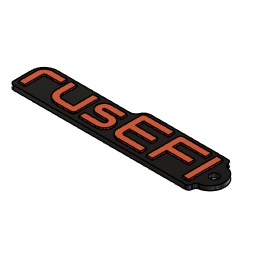
rusEFI Key chain v7 (Autodesk Fusion 360 design; units mm, degrees)
Autodesk Fusion 360 part; units mm, degrees
note: some values were not read from the file. Chosen so that the rebuilt part matches the saved one: which bodies a step acts on.
sketch "Sketch1" plane through (0, 0, 0) normal (0, 0, 1) x (1, 0, 0)
  line L0 (13.2775, 11.4505) -> (5.1185, 11.4505)
  spline S0 degree 2 poles (5.1185, 11.4505) (4.3794, 11.4505) (4.0028, 11.0809) knots 0 0 0 1 1 1
  spline S1 degree 2 poles (4.0028, 11.0809) (3.6262, 10.7113) (3.6262, 10) knots 0 0 0 1 1 1
  line L1 (3.6262, 10) -> (3.6262, 0)
  line L2 (3.6262, 0) -> (0, 0)
  line L3 (0, 0) -> (0, 10)
  spline S2 degree 2 poles (0, 10) (0, 10.9344) (0.2371, 11.6736) knots 0 0 0 1 1 1
  spline S3 degree 2 poles (0.2371, 11.6736) (0.4742, 12.4128) (0.8717, 12.9777) knots 0 0 0 1 1 1
  spline S4 degree 2 poles (0.8717, 12.9777) (1.2692, 13.5425) (1.7852, 13.94) knots 0 0 0 1 1 1
  spline S5 degree 2 poles (1.7852, 13.94) (2.3013, 14.3375) (2.8661, 14.5886) knots 0 0 0 1 1 1
  spline S6 degree 2 poles (2.8661, 14.5886) (3.431, 14.8396) (4.0098, 14.9582) knots 0 0 0 1 1 1
  spline S7 degree 2 poles (4.0098, 14.9582) (4.5886, 15.0767) (5.0907, 15.0767) knots 0 0 0 1 1 1
  line L4 (5.0907, 15.0767) -> (13.2775, 15.0767)
  line L5 (13.2775, 15.0767) -> (13.2775, 11.4505)
  spline S8 degree 2 poles (32.1478, 1.8271) (32.1478, 1.4365) (32.0084, 1.1018) knots 0 0 0 1 1 1
  spline S9 degree 2 poles (32.0084, 1.1018) (31.8689, 0.7671) (31.6248, 0.523) knots 0 0 0 1 1 1
  spline S10 degree 2 poles (31.6248, 0.523) (31.3808, 0.2789) (31.053, 0.1395) knots 0 0 0 1 1 1
  spline S11 degree 2 poles (31.053, 0.1395) (30.7252, 0) (30.3487, 0) knots 0 0 0 1 1 1
  line L6 (30.3487, 0) -> (22.1478, 0)
  spline S12 degree 2 poles (22.1478, 0) (21.4784, 0) (20.7183, 0.1534) knots 0 0 0 1 1 1
  spline S13 degree 2 poles (20.7183, 0.1534) (19.9582, 0.3068) (19.219, 0.6485) knots 0 0 0 1 1 1
  spline S14 degree 2 poles (19.219, 0.6485) (18.4798, 0.9902) (17.7894, 1.5132) knots 0 0 0 1 1 1
  spline S15 degree 2 poles (17.7894, 1.5132) (17.099, 2.0363) (16.583, 2.7824) knots 0 0 0 1 1 1
  spline S16 degree 2 poles (16.583, 2.7824) (16.0669, 3.5286) (15.7531, 4.5049) knots 0 0 0 1 1 1
  spline S17 degree 2 poles (15.7531, 4.5049) (15.4393, 5.4812) (15.4393, 6.7085) knots 0 0 0 1 1 1
  line L7 (15.4393, 6.7085) -> (15.4393, 15.0767)
  line L8 (15.4393, 15.0767) -> (19.0656, 15.0767)
  line L9 (19.0656, 15.0767) -> (19.0656, 6.7085)
  spline S18 degree 2 poles (19.0656, 6.7085) (19.0656, 5.9972) (19.3096, 5.4324) knots 0 0 0 1 1 1
  spline S19 degree 2 poles (19.3096, 5.4324) (19.5537, 4.8675) (19.9721, 4.463) knots 0 0 0 1 1 1
  spline S20 degree 2 poles (19.9721, 4.463) (20.3905, 4.0586) (20.9554, 3.8424) knots 0 0 0 1 1 1
  spline S21 degree 2 poles (20.9554, 3.8424) (21.5202, 3.6262) (22.1757, 3.6262) knots 0 0 0 1 1 1
  line L10 (22.1757, 3.6262) -> (28.5216, 3.6262)
  line L11 (28.5216, 3.6262) -> (28.5216, 15.0767)
  line L12 (28.5216, 15.0767) -> (32.1478, 15.0767)
  line L13 (32.1478, 15.0767) -> (32.1478, 1.8271)
  spline S22 degree 2 poles (50.1255, 5.0907) (50.1255, 4.1562) (49.8884, 3.41) knots 0 0 0 1 1 1
  spline S23 degree 2 poles (49.8884, 3.41) (49.6513, 2.6639) (49.2608, 2.099) knots 0 0 0 1 1 1
  spline S24 degree 2 poles (49.2608, 2.099) (48.8703, 1.5342) (48.3543, 1.1367) knots 0 0 0 1 1 1
  spline S25 degree 2 poles (48.3543, 1.1367) (47.8382, 0.7392) (47.2734, 0.4881) knots 0 0 0 1 1 1
  spline S26 degree 2 poles (47.2734, 0.4881) (46.7085, 0.2371) (46.1297, 0.1186) knots 0 0 0 1 1 1
  spline S27 degree 2 poles (46.1297, 0.1186) (45.5509, 0) (45.0349, 0) knots 0 0 0 1 1 1
  line L14 (45.0349, 0) -> (35.2162, 0)
  line L15 (35.2162, 0) -> (35.2162, 3.6262)
  line L16 (35.2162, 3.6262) -> (45.007, 3.6262)
  spline S28 degree 2 poles (45.007, 3.6262) (45.7462, 3.6262) (46.1227, 4.0028) knots 0 0 0 1 1 1
  spline S29 degree 2 poles (46.1227, 4.0028) (46.4993, 4.3794) (46.4993, 5.0907) knots 0 0 0 1 1 1
  spline S30 degree 2 poles (46.4993, 5.0907) (46.4296, 6.5411) (45.0349, 6.5411) knots 0 0 0 1 1 1
  line L17 (45.0349, 6.5411) -> (39.4142, 6.5411)
  spline S31 degree 2 poles (39.4142, 6.5411) (38.2148, 6.5411) (37.378, 6.9596) knots 0 0 0 1 1 1
  spline S32 degree 2 poles (37.378, 6.9596) (36.5411, 7.378) (36.0181, 8.0056) knots 0 0 0 1 1 1
  spline S33 degree 2 poles (36.0181, 8.0056) (35.4951, 8.6332) (35.265, 9.3584) knots 0 0 0 1 1 1
  spline S34 degree 2 poles (35.265, 9.3584) (35.0349, 10.0837) (35.0349, 10.7113) knots 0 0 0 1 1 1
  spline S35 degree 2 poles (35.0349, 10.7113) (35.0349, 11.9247) (35.4672, 12.7545) knots 0 0 0 1 1 1
  spline S36 degree 2 poles (35.4672, 12.7545) (35.8996, 13.5844) (36.5551, 14.1004) knots 0 0 0 1 1 1
  spline S37 degree 2 poles (36.5551, 14.1004) (37.2106, 14.6165) (37.9777, 14.8466) knots 0 0 0 1 1 1
  spline S38 degree 2 poles (37.9777, 14.8466) (38.7448, 15.0767) (39.4142, 15.0767) knots 0 0 0 1 1 1
  line L18 (39.4142, 15.0767) -> (48.3264, 15.0767)
  line L19 (48.3264, 15.0767) -> (48.3264, 11.4505)
  line L20 (48.3264, 11.4505) -> (39.4421, 11.4505)
  spline S39 degree 2 poles (39.4421, 11.4505) (39.1632, 11.4505) (39.0028, 11.3877) knots 0 0 0 1 1 1
  spline S40 degree 2 poles (39.0028, 11.3877) (38.8424, 11.325) (38.7657, 11.2204) knots 0 0 0 1 1 1
  spline S41 degree 2 poles (38.7657, 11.2204) (38.689, 11.1158) (38.675, 10.9972) knots 0 0 0 1 1 1
  spline S42 degree 2 poles (38.675, 10.9972) (38.6611, 10.8787) (38.6611, 10.7671) knots 0 0 0 1 1 1
  spline S43 degree 2 poles (38.6611, 10.7671) (38.675, 10.5439) (38.7448, 10.4184) knots 0 0 0 1 1 1
  spline S44 degree 2 poles (38.7448, 10.4184) (38.8145, 10.2929) (38.9191, 10.2371) knots 0 0 0 1 1 1
  spline S45 degree 2 poles (38.9191, 10.2371) (39.0237, 10.1813) (39.1562, 10.1743) knots 0 0 0 1 1 1
  spline S46 degree 2 poles (39.1562, 10.1743) (39.2887, 10.1674) (39.4142, 10.1674) knots 0 0 0 1 1 1
  line L21 (39.4142, 10.1674) -> (45.0349, 10.1674)
  spline S47 degree 2 poles (45.0349, 10.1674) (46.4296, 10.1674) (47.4059, 9.6653) knots 0 0 0 1 1 1
  spline S48 degree 2 poles (47.4059, 9.6653) (48.3821, 9.1632) (48.9819, 8.4031) knots 0 0 0 1 1 1
  spline S49 degree 2 poles (48.9819, 8.4031) (49.5816, 7.643) (49.8536, 6.7504) knots 0 0 0 1 1 1
  spline S50 degree 2 poles (49.8536, 6.7504) (50.1255, 5.8577) (50.1255, 5.0907) knots 0 0 0 1 1 1
  line L22 (69.5119, 8.1729) -> (56.6109, 8.1729)
  line L23 (56.6109, 11.8271) -> (69.5119, 11.8271)
  line L24 (69.5119, 11.8271) -> (69.5119, 8.1729)
  line L25 (71.1437, 0) -> (58.0614, 0)
  spline S51 degree 2 poles (58.0614, 0) (57.3082, 0) (56.4156, 0.265) knots 0 0 0 1 1 1
  spline S52 degree 2 poles (56.4156, 0.265) (55.523, 0.53) (54.7629, 1.1367) knots 0 0 0 1 1 1
  spline S53 degree 2 poles (54.7629, 1.1367) (54.0028, 1.7434) (53.4937, 2.7127) knots 0 0 0 1 1 1
  spline S54 degree 2 poles (53.4937, 2.7127) (52.9847, 3.682) (52.9847, 5.0907) knots 0 0 0 1 1 1
  line L26 (52.9847, 5.0907) -> (52.9847, 18.1729)
  spline S55 degree 2 poles (52.9847, 18.1729) (52.9847, 18.5495) (53.1241, 18.8842) knots 0 0 0 1 1 1
  spline S56 degree 2 poles (53.1241, 18.8842) (53.2636, 19.219) (53.5077, 19.47) knots 0 0 0 1 1 1
  spline S57 degree 2 poles (53.5077, 19.47) (53.7517, 19.7211) (54.0865, 19.8605) knots 0 0 0 1 1 1
  spline S58 degree 2 poles (54.0865, 19.8605) (54.4212, 20) (54.8117, 20) knots 0 0 0 1 1 1
  line L27 (54.8117, 20) -> (71.1437, 20)
  line L28 (71.1437, 20) -> (71.1437, 16.3738)
  line L29 (71.1437, 16.3738) -> (56.6109, 16.3738)
  spline S59 degree 2 poles (56.6109, 5.0907) (56.6109, 4.3794) (56.9874, 4.0028) knots 0 0 0 1 1 1
  spline S60 degree 2 poles (56.9874, 4.0028) (57.364, 3.6262) (58.0893, 3.6262) knots 0 0 0 1 1 1
  line L30 (58.0893, 3.6262) -> (71.1437, 3.6262)
  line L31 (71.1437, 3.6262) -> (71.1437, 0)
  line L32 (91.1855, 8.1729) -> (78.2706, 8.1729)
  line L33 (78.2706, 11.8271) -> (91.1855, 11.8271)
  line L34 (91.1855, 11.8271) -> (91.1855, 8.1729)
  line L35 (92.8034, 16.3738) -> (78.2706, 16.3738)
  line L36 (78.2706, 0) -> (74.6444, 0)
  line L37 (74.6444, 0) -> (74.6444, 18.1729)
  spline S61 degree 2 poles (74.6444, 18.1729) (74.6444, 18.5495) (74.7838, 18.8842) knots 0 0 0 1 1 1
  spline S62 degree 2 poles (74.7838, 18.8842) (74.9233, 19.219) (75.1674, 19.47) knots 0 0 0 1 1 1
  spline S63 degree 2 poles (75.1674, 19.47) (75.4114, 19.7211) (75.7462, 19.8605) knots 0 0 0 1 1 1
  spline S64 degree 2 poles (75.7462, 19.8605) (76.0809, 20) (76.4714, 20) knots 0 0 0 1 1 1
  line L38 (76.4714, 20) -> (92.8034, 20)
  line L39 (92.8034, 20) -> (92.8034, 16.3738)
  line L40 (99.3863, 0) -> (95.7601, 0)
  line L41 (95.7601, 0) -> (95.7601, 20)
  line L42 (95.7601, 20) -> (99.3863, 20)
  line L43 (99.3863, 20) -> (99.3863, 0)
  line L44 (56.6109, 16.3738) -> (56.6109, 11.8271)
  line L45 (56.6109, 8.1729) -> (56.6109, 5.0907)
  line L46 (78.2706, 16.3738) -> (78.2706, 11.8271)
  line L47 (78.2706, 8.1729) -> (78.2706, 0)
  constraint coincident L22.end L44
  constraint coincident L32.end L46
  constraint collinear L44 L45
  constraint collinear L46 L47
sketch "Sketch4" plane through (0, 0, 0) normal (0, 0, 1) x (1, 0, 0)
  line L0 (8.6262, 17.5767) -> (10.4393, 17.5767)
  line L1 (10.4393, 17.5767) -> (18.2775, 17.5767)
  line L2 (18.2775, 17.5767) -> (24.0656, 17.5767)
  line L3 (24.0656, 17.5767) -> (37.1478, 17.5767)
  line L4 (37.1478, 17.5767) -> (47.763, 17.5767)
  spline S0 degree 3 poles (50.8164, 19.8458) (51.0141, 20.3201) (51.3471, 20.8341) (51.7152, 21.2127) knots 0 0 0 0 0.999986 0.999986 0.999986 0.999986
  spline S1 degree 3 poles (51.7152, 21.2127) (52.0946, 21.603) (52.6372, 21.965) (53.1249, 22.1682) knots 0 0 0 0 0.99999 0.99999 0.99999 0.99999
  spline S2 degree 3 poles (53.1249, 22.1682) (53.6457, 22.3852) (54.2787, 22.5) (54.8117, 22.5) knots 0 0 0 0 1 1 1 1
  line L5 (54.8117, 22.5) -> (90.7601, 22.5)
  line L6 (90.7601, 22.5) -> (97.8034, 22.5)
  line L7 (97.8034, 22.5) -> (99.8863, 22.5)
  line L8 (101.8863, 20.5) -> (101.8863, -0.5)
  line L9 (99.8863, -2.5) -> (93.2601, -2.5)
  line L10 (80.7706, -2.5) -> (76.1437, -2.5)
  line L11 (76.1437, -2.5) -> (69.6444, -2.5)
  line L12 (69.6444, -2.5) -> (58.0614, -2.5)
  spline S3 degree 3 poles (58.0614, -2.5) (57.2575, -2.5) (56.4899, -2.3649) (55.7041, -2.1316) knots 0 0 0 0 1 1 1 1
  spline S4 degree 3 poles (55.7041, -2.1316) (54.8116, -1.8667) (53.931, -1.398) (53.2034, -0.8172) knots 0 0 0 0 1 1 1 1
  spline S5 degree 3 poles (49.8798, -0.8439) (49.6352, -1.0323) (49.3782, -1.208) (49.1119, -1.3678) (48.9742, -1.4504) (48.834, -1.5288) (48.6918, -1.6025) (48.5907, -1.6549) (48.4885, -1.705) (48.3854, -1.7526) (48.3533, -1.7674) (48.3103, -1.7868) (48.2887, -1.7964) knots 0.000003 0.000003 0.000003 0.000003 0.500008 0.500008 0.500008 0.758594 0.758594 0.758594 0.942579 0.942579 0.942579 1.000013 1.000013 1.000013 1.000013
  spline S6 degree 3 poles (48.2887, -1.7964) (47.7583, -2.0321) (47.1981, -2.2145) (46.6314, -2.3306) knots 0.000004 0.000004 0.000004 0.000004 0.999993 0.999993 0.999993 0.999993
  spline S7 degree 3 poles (46.6314, -2.3306) (46.5732, -2.3425) (46.4714, -2.3623) (46.3915, -2.3764) (45.941, -2.4562) (45.4914, -2.5) (45.0349, -2.5) knots -0.000019 -0.000019 -0.000019 -0.000019 0.150705 0.150705 0.150705 1 1 1 1
  line L13 (45.0349, -2.5) -> (30.3487, -2.5)
  line L14 (30.3487, -2.5) -> (30.2162, -2.5)
  line L15 (30.2162, -2.5) -> (22.1478, -2.5)
  line L16 (6.1262, -2.5) -> (-0.5, -2.5)
  line L17 (-2.5, -0.5) -> (-2.5, 10)
  spline S8 degree 3 poles (-2.5, 10) (-2.5, 10.8374) (-2.3964, 11.6486) (-2.1434, 12.4372) knots 0 0 0 0 0.999997 0.999997 0.999997 0.999997
  spline S9 degree 3 poles (-2.1434, 12.4372) (-1.919, 13.1368) (-1.5967, 13.8141) (-1.1728, 14.4164) knots 0 0 0 0 0.999995 0.999995 0.999995 0.999995
  spline S10 degree 3 poles (-1.1728, 14.4164) (-0.7781, 14.9773) (-0.2862, 15.5002) (0.2596, 15.9206) knots 0 0 0 0 1 1 1 1
  spline S11 degree 3 poles (0.2596, 15.9206) (0.7488, 16.2974) (1.2879, 16.6229) (1.8508, 16.8731) knots 0 0 0 0 1 1 1 1
  spline S12 degree 3 poles (1.8508, 16.8731) (2.3812, 17.1088) (2.9414, 17.2912) (3.5081, 17.4073) knots 0 0 0 0 0.999995 0.999995 0.999995 0.999995
  spline S13 degree 3 poles (3.5081, 17.4073) (4.0368, 17.5156) (4.5551, 17.5767) (5.0907, 17.5767) knots 0 0 0 0 1 1 1 1
  line L18 (5.0907, 17.5767) -> (8.6262, 17.5767)
  line L19 (22.1478, -2.5) -> (6.1262, -2.5)
  line L20 (80.7706, -2.5) -> (93.2601, -2.5)
  arc A0 (53.2034, -0.8172) -> (49.8798, -0.8439) centre (51.5592, -3.0241) ccw
  arc A1 (47.763, 17.5767) -> (50.8164, 19.8458) centre (47.3837, 21.2761) ccw
  line L21 (45.0349, -2.5) -> (58.0614, -2.5)
  arc A2 (99.8863, -2.5) -> (101.8863, -0.5) centre (99.8863, -0.5) ccw
  arc A3 (101.8863, 20.5) -> (99.8863, 22.5) centre (99.8863, 20.5) ccw
  arc A4 (-2.5, -0.5) -> (-0.5, -2.5) centre (-0.5, -0.5) ccw
  dimension "d24" = 2
  dimension "d25" = 2
  dimension "d28" = 2
  constraint tangent S5 A0
  constraint tangent S0 A1
  constraint tangent L8 A2
  constraint tangent L9 A2
  constraint tangent L7 A3
  constraint tangent L8 A3
  constraint tangent L16 A4
  constraint tangent L17 A4
  measures "d24" radius of A2
  measures "d25" radius of A3
  measures "d28" radius of A4
extrude "Extrude2" add sketch "Sketch4" along normal blind 2.5 makes body 1
extrude "Extrude3" add sketch "Sketch1" along normal blind 3.5 separate body makes body 2 at (75.8531, 8.782, 0) makes body 3 at (30.9391, 6.8433, 0) makes body 4 at (41.7527, 1.2087, 0) makes body 5 at (1.2087, 6.6667, 0) makes body 6 at (54.1934, 11.6969, 0) makes body 7 at (96.9689, 6.6667, 0)
split "Split1" by plane through (0, 0, 2.5) normal (0, 0, 1) bodies 7 6 3 5 4 2 makes body 10 at (75.8531, 8.782, 3.5) makes body 12 at (41.7527, 1.2087, 3.5) makes body 11 at (1.2087, 6.6667, 3.5) makes body 9 at (30.9391, 6.8433, 3.5) makes body 13 at (54.1934, 11.6969, 3.5) makes body 8 at (96.9689, 6.6667, 3.5)
sketch "Sketch5" plane through (0, 0, 0) normal (0, 0, 1) x (1, 0, 0)
  line L0 (101.8863, 20.5) -> (101.8863, -0.5)
  arc A0 (103.6562, 1.6863) -> (110.3863, 10) centre (101.8863, 10) ccw
  arc A1 (101.8863, 5) -> (101.8863, 15) centre (101.8863, 10) ccw construction
  arc A2 (103.6562, 1.6863) -> (101.8863, -0.5) centre (104.1216, -0.5) ccw
  circle A3 centre (104.3863, 10) radius 2.5
  line L1 (110.3863, 10) -> (101.8863, 10)
  arc A4 (110.3863, 10) -> (103.6562, 18.3137) centre (101.8863, 10) ccw
  arc A5 (101.8863, 20.5) -> (103.6562, 18.3137) centre (104.1216, 20.5) ccw
  dimension "d14" = 10
  dimension "d23" = 5
  constraint midpoint A0.centre L0
  constraint concentric A0 A1
  constraint coincident L0 A1.end
  constraint coincident L0 A1.start
  constraint tangent L0 A2
  constraint tangent A0 A2
  constraint coincident L0.end A2.end
  constraint coincident A0.centre A3
  constraint coincident A0.centre A1.centre
  constraint perpendicular L0 L1
  constraint symmetric A0 L1 A4
  constraint symmetric A0.start L1 A4.end
  constraint symmetric L0.end L1 L0.start
  constraint symmetric A2 L1 A5
  constraint symmetric A0.end L1 A4.start
  measures "d14" diameter of A1
  measures "d23" diameter of A3
extrude "Extrude6" add sketch "Sketch5" along normal up to surface (2.5 mm away) contours L0 A3 L1 A4 A5 | L0 A0 A2 A3 L1 bodies 1
hidden bodies 6 5 2 4 3 7
